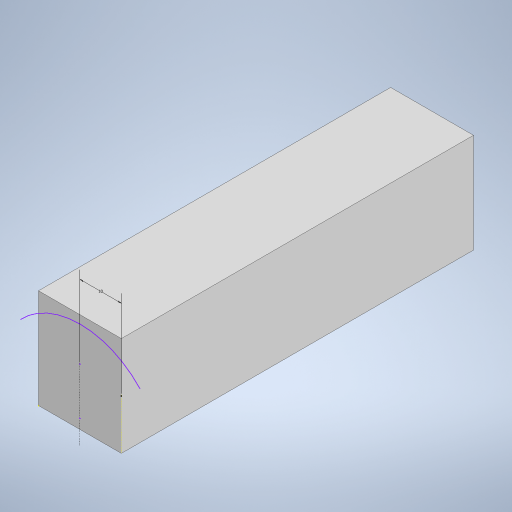
# Autodesk Inventor part: Modulo lectura
Saved by Autodesk Inventor 2023 (Build 270158000, 158)
## iProperties
Created: 2022-07-15
Part Number: Modulo lectura
Material: Genérico
Document SubType Name: Modeling
Designer: juand
Density: 1 g/cm^3
Appearance: Valor por defecto
Author: juand
Autodesk Inventor part; units mm, degrees
ref_plane "YZ Plane" through (0, 0, 0) normal (1, 0, 0) x (0, 1, 0)
ref_plane "XZ Plane" through (0, 0, 0) normal (0, 1, 0) x (-1, 0, 0)
ref_plane "XY Plane" through (0, 0, 0) normal (0, 0, 1) x (1, 0, 0)
sketch "Boceto1" plane through (0, 0, 0) normal (0, 1, 0) x (-1, 0, 0)
  line L0 (-20, 0) -> (0, 0)
  line L1 (0, 0) -> (0, 85)
  line L2 (0, 85) -> (-20, 85)
  line L3 (-20, 85) -> (-20, 0)
  dimension "d0" = 85
  dimension "d1" = 20
  constraints: 8 end point, 2 parallel, 2 point on line, 1 horizontal, 1 perpendicular
  measures "d0" distance of L0.end L1.end
  measures "d1" distance of L1.end L2.end
extrude "Extrusión1" add sketch "Boceto1" along normal blind 24
sketch "Boceto2" plane through (0, 0, 85) normal (0, 0, 1) x (1, 0, 0)
  arc A0 (24.444, 15.7821) -> (-4.444, 15.7821) centre (10, 2.3061) ccw
  line L0 (10, 30.8468) -> (10, -3.4075) construction
  line L1 (20, 0) -> (20, 24) construction
  point P0 (0, 0)
  point P1 (20, 12)
  point P2 (10, 13.7196)
  dimension "d4" = 10
  constraints: 2 end point, 2 midpoint, 2 point on circle, 1 centre point, 1 symmetric about line, 1 vertical
  measures "d4" horizontal distance of point (20, 12) point (10, 13.72)
